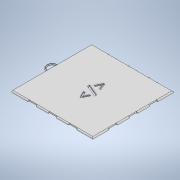
# Autodesk Inventor part: Back
Saved by Autodesk Inventor 2020 (Build 240168000, 168)
## iProperties
Created: 2020-06-10
Part Number: Back
Material: Generic
Document SubType Name: Modeling
Designer: maple
Density: 1 g/cm^3
Appearance: Default
Author: maple
Autodesk Inventor part; units mm, degrees
ref_plane "YZ Plane" through (0, 0, 0) normal (1, 0, 0) x (0, 1, 0)
ref_plane "XZ Plane" through (0, 0, 0) normal (0, 1, 0) x (-1, 0, 0)
ref_plane "XY Plane" through (0, 0, 0) normal (0, 0, 1) x (1, 0, 0)
sketch "Sketch1" plane through (0, 0, 0) normal (0, 1, 0) x (-1, 0, 0)
  line L0 (0, 0) -> (-100, 0)
  line L1 (-100, 0) -> (-100, -100)
  line L2 (-100, -100) -> (0, -100)
  line L3 (0, -100) -> (0, 0)
  line L4 (-100, 0) -> (-100, -25)
  line L5 (-100, -25) -> (-100, -50)
  line L6 (-100, -50) -> (-100, -75)
  line L7 (-100, 0) -> (-75, 0)
  line L8 (-75, 0) -> (-50, 0)
  line L9 (-50, 0) -> (-25, 0)
  line L10 (-75, 0) -> (-80, 0)
  line L11 (-50, 0) -> (-55, 0)
  line L12 (-25, 0) -> (-30, 0)
  line L13 (-100, -25) -> (-100, -20)
  line L14 (-100, -50) -> (-100, -45)
  line L15 (-100, -75) -> (-100, -70)
  line L16 (-80, 0) -> (-70, 0)
  line L17 (-70, 0) -> (-70, -1.5)
  line L18 (-70, -1.5) -> (-80, -1.5)
  line L19 (-80, -1.5) -> (-80, 0)
  line L20 (-55, 0) -> (-45, 0)
  line L21 (-45, 0) -> (-45, -1.5)
  line L22 (-45, -1.5) -> (-55, -1.5)
  line L23 (-55, -1.5) -> (-55, 0)
  line L24 (-30, 0) -> (-20, 0)
  line L25 (-20, 0) -> (-20, -1.5)
  line L26 (-20, -1.5) -> (-30, -1.5)
  line L27 (-30, -1.5) -> (-30, 0)
  line L28 (-100, -20) -> (-98.5, -20)
  line L29 (-98.5, -20) -> (-98.5, -30)
  line L30 (-98.5, -30) -> (-100, -30)
  line L31 (-100, -30) -> (-100, -20)
  line L32 (-100, -45) -> (-98.5, -45)
  line L33 (-98.5, -45) -> (-98.5, -55)
  line L34 (-98.5, -55) -> (-100, -55)
  line L35 (-100, -55) -> (-100, -45)
  line L36 (-100, -70) -> (-98.5, -70)
  line L37 (-98.5, -70) -> (-98.5, -80)
  line L38 (-98.5, -80) -> (-100, -80)
  line L39 (-100, -80) -> (-100, -70)
  line L40 (-80, -100) -> (-70, -100)
  line L41 (-70, -100) -> (-70, -98.5)
  line L42 (-70, -98.5) -> (-80, -98.5)
  line L43 (-80, -98.5) -> (-80, -100)
  line L44 (-55, -100) -> (-45, -100)
  line L45 (-45, -100) -> (-45, -98.5)
  line L46 (-45, -98.5) -> (-55, -98.5)
  line L47 (-55, -98.5) -> (-55, -100)
  line L48 (-30, -100) -> (-20, -100)
  line L49 (-20, -100) -> (-20, -98.5)
  line L50 (-20, -98.5) -> (-30, -98.5)
  line L51 (-30, -98.5) -> (-30, -100)
  line L52 (0, -50) -> (0, -57)
  circle A0 centre (0, -50) radius 7
  line L53 (0, -57) -> (0, -55)
  circle A1 centre (0, -50) radius 5
  point P0 (0, -43)
  point P1 (0, -45)
  dimension "d0" = 100
  dimension "d1" = 100
  dimension "d2" = 25
  dimension "d3" = 25
  dimension "d4" = 25
  dimension "d5" = 25
  dimension "d6" = 25
  dimension "d7" = 25
  dimension "d8" = 5
  dimension "d9" = 5
  dimension "d10" = 5
  dimension "d11" = 5
  dimension "d12" = 5
  dimension "d13" = 5
  dimension "d14" = 10
  dimension "d15" = 1.5
  dimension "d16" = 10
  dimension "d17" = 1.5
  dimension "d18" = 10
  dimension "d19" = 1.5
  dimension "d20" = 1.5
  dimension "d21" = 10
  dimension "d22" = 1.5
  dimension "d23" = 10
  dimension "d24" = 1.5
  dimension "d25" = 10
  dimension "d26" = 10
  dimension "d27" = 1.5
  dimension "d28" = 10
  dimension "d29" = 1.5
  dimension "d30" = 10
  dimension "d31" = 1.5
  dimension "d35" = 7
  dimension "d36" = 2
  constraints: 108 end point, 20 parallel, 18 point on line, 10 horizontal, 10 perpendicular, 3 midpoint, 2 coincident, 6 other
  measures "d0" distance of L2.end L1.end
  measures "d1" distance of L1.end L0.end
  measures "d2" distance of L0.end L4.end
  measures "d3" distance of L4.end L5.end
  measures "d4" distance of L5.end L6.end
  measures "d5" distance of L0.end L7.end
  measures "d6" distance of L7.end L8.end
  measures "d7" distance of L8.end L9.end
  measures "d8" distance of L7.end L10.end
  measures "d9" distance of L8.end L11.end
  measures "d10" distance of L9.end L12.end
  measures "d11" distance of L4.end L13.end
  measures "d12" distance of L5.end L14.end
  measures "d13" distance of L6.end L15.end
  measures "d14" distance of L17.end L18.end
  measures "d15" distance of L16.end L17.end
  measures "d16" distance of L21.end L22.end
  measures "d17" distance of L20.end L21.end
  measures "d18" distance of L25.end L26.end
  measures "d19" distance of L24.end L25.end
  measures "d20" distance of L29.end L30.end
  measures "d21" distance of L28.end L29.end
  measures "d22" distance of L33.end L34.end
  measures "d23" distance of L32.end L33.end
  measures "d24" distance of L37.end L38.end
  measures "d25" distance of L36.end L37.end
  measures "d26" distance of L42.end L41.end
  measures "d27" distance of L41.end L40.end
  measures "d28" distance of L46.end L45.end
  measures "d29" distance of L45.end L44.end
  measures "d30" distance of L50.end L49.end
  measures "d31" distance of L49.end L48.end
  measures "d35" distance of L52.start L52.end
  measures "d36" distance of L52.end L53.end
extrude "Extrusion1" add sketch "Sketch1" along normal blind 1.5 contours L3 A0 L2 L49 L50 L51 L45 L46 L47 L41 L42 L43 L1 L38 L37 L36 L34 L33 L32 L30 L29 L28 L0 L19 L18 L17 L23 L22 L21 L27 L26 L25 | A0 L3 A1 | L3 A1 A0 | L3 A1 picked at (-0.3989, -53.2849)
fillet "Fillet1" radius 1.5 12 edges at (10, 1.5, 0) (37.5, 1.5, 0) (62.5, 1.5, 0) (90, 1.5, 0) (100, 1.5, -10) (100, 1.5, -37.5) (100, 1.5, -62.5) (100, 1.5, -90) (90, 1.5, -100) (62.5, 1.5, -100) (37.5, 1.5, -100) (10, 1.5, -100)
fillet "Fillet2" radius 0.8 4 edges at (-5, 1.5, -50) (-7, 1.5, -50) (-7, 0, -50) (-5, 0, -50)
sketch "Sketch2" plane through (0, 1.5, 0) normal (0, 1, 0) x (1, 0, 0)
  line L0 (0, 55.8) -> (0, 44.2) projected
  line L1 (0, 50) -> (98.5, 50)
  line L2 (98.5, 45) -> (98.5, 55) projected
  line L3 (47.3935, 45.7714) -> (47.3935, 54.1978) construction
  line L4 (47.3935, 54.1978) -> (51.0957, 54.1978) construction
  line L5 (51.0957, 54.1978) -> (51.0957, 45.7714) construction
  line L6 (51.0957, 45.7714) -> (47.3935, 45.7714) construction
  line L7 (53.9864, 43.6876) -> (50.2047, 35.4173)
  line L8 (50.2047, 35.4173) -> (48.7674, 35.4173)
  line L9 (48.7674, 35.4173) -> (44.809, 43.6876)
  line L10 (44.809, 43.6876) -> (46.9178, 43.6876)
  line L11 (46.9178, 43.6876) -> (49.4507, 37.7971)
  line L12 (49.4507, 37.7971) -> (49.4979, 37.7971)
  line L13 (49.4979, 37.7971) -> (51.8776, 43.6876)
  line L14 (51.8776, 43.6876) -> (53.9864, 43.6876)
  line L15 (41.8402, 54.2199) -> (56.649, 48.023)
  line L16 (56.649, 48.023) -> (56.649, 45.5254)
  line L17 (56.649, 45.5254) -> (41.8402, 51.6987)
  line L18 (41.8402, 51.6987) -> (41.8402, 54.2199)
  line L19 (50.0987, 64.5637) -> (53.8686, 56.2933)
  line L20 (53.8686, 56.2933) -> (51.7716, 56.2933)
  line L21 (51.7716, 56.2933) -> (49.4036, 62.2074)
  line L22 (49.4036, 62.2074) -> (49.3683, 62.2074)
  line L23 (49.3683, 62.2074) -> (46.8353, 56.2933)
  line L24 (46.8353, 56.2933) -> (44.7265, 56.2933)
  line L25 (44.7265, 56.2933) -> (48.6614, 64.5637)
  line L26 (48.6614, 64.5637) -> (50.0987, 64.5637)
  point P0 (0, 0)
  point P1 (49.25, 50)
  constraints: 3 midpoint, 2 end point, 2 other
emboss "Emboss1" sketch "Sketch2" operation cut depth 1.5 direction (0, -1, 0)
body "Solid1"
